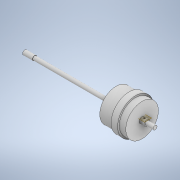
# Autodesk Inventor part: ellensuly
Saved by Autodesk Inventor 2021.4 (Build 254397000, 397)
## iProperties
Created: 2023-12-02
Part Number: ellensuly
Material: Generic
Document SubType Name: Modeling
Designer: vtoth
Density: 1 g/cm^3
Appearance: Default
Author: vtoth
Autodesk Inventor part; units mm, degrees
ref_plane "YZ Plane" through (0, 0, 0) normal (1, 0, 0) x (0, 1, 0)
ref_plane "XZ Plane" through (0, 0, 0) normal (0, 1, 0) x (-1, 0, 0)
ref_plane "XY Plane" through (0, 0, 0) normal (0, 0, 1) x (1, 0, 0)
sketch "Sketch1" plane through (0, 0, 0) normal (0, 0, 1) x (1, 0, 0)
  line L0 (0, 66) -> (0, -11) construction
  line L1 (-80, 0) -> (480, 0) construction
  line L2 (0, 0) -> (0, 7)
  line L3 (0, 7) -> (30, 7)
  line L4 (30, 7) -> (30, 6)
  line L5 (30, 6) -> (400, 6)
  line L6 (400, 6) -> (400, 0)
  line L7 (0, 0) -> (400, 0)
  line L8 (280, 6) -> (280, 50)
  line L9 (280, 50) -> (320, 50)
  line L10 (320, 50) -> (320, 55)
  line L11 (320, 55) -> (340, 55)
  line L12 (340, 55) -> (340, 50)
  line L13 (340, 50) -> (360, 50)
  line L14 (360, 50) -> (360, 9)
  line L15 (360, 9) -> (375, 9)
  line L16 (375, 9) -> (375, 6)
  point P0 (367.5, 9)
  dimension "d0" = 14
  dimension "d1" = 12
  dimension "d2" = 30
  dimension "d3" = 400
  dimension "d4" = 80
  dimension "d5" = 15
  dimension "d6" = 20
  dimension "d7" = 40
  dimension "d8" = 110
  dimension "d9" = 100
  dimension "d10" = 25
  dimension "d11" = 3
  constraints: 30 end point, 10 perpendicular, 6 point on line, 3 vertical, 2 collinear, 1 coincident, 1 midpoint
  measures "d0" diameter of L3 L1
  measures "d1" diameter of L5 L1
  measures "d2" distance between parallel lines of L4 L2
  measures "d3" distance between parallel lines of L6 L2
  measures "d4" distance between parallel lines of L14 L8
  measures "d5" distance between parallel lines of L16 L14
  measures "d6" distance between parallel lines of L12 L10
  measures "d7" distance between parallel lines of L8 L10
  measures "d8" diameter of L11 L1
  measures "d9" diameter of L9 L1
  measures "d10" distance between parallel lines of L6 L16
  measures "d11" distance between parallel lines of L5 L15
revolve "Revolution1" add sketch "Sketch1" angle 360 about axis through (0, 0, 0) along (1, 0, 0) contours L2 L3 L4 L5 L6 L7
revolve "Revolution2" add sketch "Sketch1" angle 360 about axis through (0, 0, 0) along (1, 0, 0) separate body contours L5 L8 L9 L10 L11 L12 L13 L14 L15 L16
ref_plane "Work Plane1" through (367.5, 9, 0) normal (0, 1, 0) x (-1, 0, 0)
sketch "Sketch2" plane through (367.5, 9, 0) normal (0, 1, 0) x (-1, 0, 0)
  point P0 (367.5, 0)
  point P1 (0, 0)
hole "Hole1" at (367.5, 9, 0) direction (0, -1, 0) diameter 4.917 end up to face face through (327.5, 0, 0) facing (1, 0, 0) round with radius 6 far side no bodies 2 thread size "M6x1" class "6H" standard "ISO Metric profile"
sketch "Sketch3" plane through (0, 0, 0) normal (-1, 0, 0) x (0, 0, 1)
  point P0 (0, 0)
  point P1 (0, 0)
hole "Hole2" at (0, 0, 0) direction (1, 0, 0) diameter 8.376 depth 27.3 tip angle 118 bodies 1 thread size "M10x1.5" class "6H" standard "ISO Metric profile"
